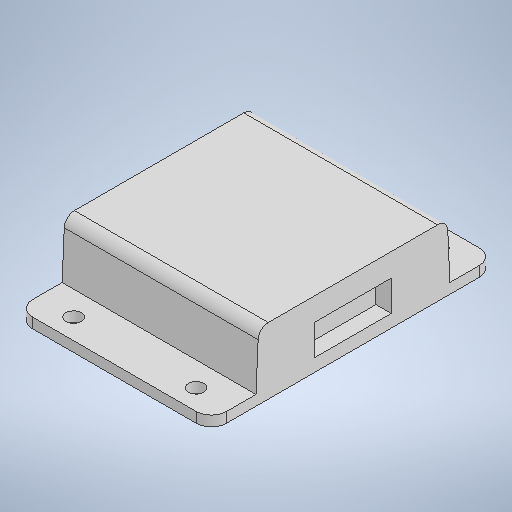
# Autodesk Inventor part: LiDAR_slave
Saved by Autodesk Inventor 2025.1 (Build 291241020, 241B)
## iProperties
Created: 2024-09-23
Part Number: LiDAR_slave
Material: 一般
Document SubType Name: Modeling
Designer: 8326d
Density: 1 g/cm^3
Appearance: 既定
Author: 8326d
Autodesk Inventor part; units mm, degrees
ref_plane "YZ Plane" through (0, 0, 0) normal (1, 0, 0) x (0, 1, 0)
ref_plane "XZ Plane" through (0, 0, 0) normal (0, 1, 0) x (-1, 0, 0)
ref_plane "XY Plane" through (0, 0, 0) normal (0, 0, 1) x (1, 0, 0)
sketch "スケッチ1" plane through (0, 0, 0) normal (1, 0, 0) x (0, 1, 0)
  line L0 (-6.5, 27.75) -> (6.5, 27.75)
  line L1 (6.5, 27.75) -> (6.5, -27.75)
  line L2 (6.5, -27.75) -> (-6.5, -27.75)
  line L3 (-6.5, -27.75) -> (-6.5, 27.75)
  line L4 (-6.5, 27.75) -> (6.5, -27.75) construction
  line L5 (6.5, 27.75) -> (-6.5, -27.75) construction
  line L6 (6.5, 19) -> (-4.5, 19)
  line L7 (-4.5, 19) -> (-4.5, -19)
  line L8 (-4.5, -19) -> (6.5, -19)
  line L9 (6.5, -19) -> (6.5, 19)
  line L10 (-4.5, 27.75) -> (-4.5, 19)
  line L11 (-4.5, 19) -> (6.5, 18.5)
  line L12 (6.5, -18.5) -> (-4.5, -19)
  line L13 (-4.5, -19) -> (-4.5, -27.75)
  point P0 (0, 0)
  point P1 (6.5, 0)
  point P2 (6.5, 18.5)
  dimension "d0" = 13
  dimension "d1" = 55.5
  dimension "d2" = 11
  dimension "d3" = 38
  dimension "d4" = 0.5
  dimension "d5" = 0.5
  constraints: 28 end point, 6 point on line, 4 midpoint, 4 parallel, 2 horizontal, 2 perpendicular, 1 collinear
  measures "d0" distance of L1.end L2.end
  measures "d1" distance of L0.end L1.end
  measures "d2" distance of L8.end L7.end
  measures "d3" distance of L7.end L6.end
  measures "d4" distance from line of L6 L11.end
  measures "d5" distance from line of L8 L12.start
extrude "押し出し1" add sketch "スケッチ1" along normal mid plane 38 contours L0 L10 L7 L13 L2 L3 | L11 L1 L12 L7
fillet "フィレット1" radius 2 2 edges at (0, 6.5, 18.5) (0, 6.5, -18.5)
sketch "スケッチ2" plane through (-19, -4.5, 27.75) normal (0, 1, 0) x (1, 0, 0)
  line L0 (7, 4) -> (31, 4) construction
  line L1 (7, 4) -> (31, 4) construction
  line L2 (0, 0) -> (38, 0) construction
  point P0 (19, 27.75)
  point P1 (19, 4)
  dimension "d9" = 24
  dimension "d10" = 0
  dimension "d11" = 4
  constraints: 4 end point, 2 coincident, 2 horizontal, 1 collinear, 1 midpoint, 1 vertical alignment
  measures "d9" distance of L0.start L0.end
  measures "d10" distance between parallel lines of L0 L1
  measures "d11" distance between parallel lines of L2 L0
hole "穴1" at (-12, -4.5, 23.75) at (12, -4.5, 23.75) direction (0, -1, 0) diameter 3 end through all
fillet "フィレット2" radius 3 2 edges at (19, -5.5, 27.75) (-19, -5.5, 27.75)
mirror "ミラー1" about plane through (0, 0, 0) normal (0, 0, 1) of "穴1", "フィレット2"
sketch "スケッチ3" plane through (19, 0, 0) normal (1, 0, 0) x (0, 0, -1)
  line L0 (-7.5, -4) -> (7.5, -4)
  line L1 (7.5, -4) -> (7.5, 2)
  line L2 (7.5, 2) -> (-7.5, 2)
  line L3 (-7.5, 2) -> (-7.5, -4)
  line L4 (-7.5, -4) -> (7.5, 2) construction
  line L5 (7.5, -4) -> (-7.5, 2) construction
  line L6 (-24.75, -6.5) -> (24.75, -6.5) projected
  point P0 (0, 0)
  point P1 (0, -1)
  dimension "d20" = 15
  dimension "d21" = 6
  dimension "d22" = 2.5
  constraints: 12 end point, 2 midpoint, 2 parallel, 1 horizontal, 1 perpendicular, 1 vertical alignment
  measures "d20" distance of L2.end L1.end
  measures "d21" distance of L1.end L0.end
  measures "d22" distance between parallel lines of L6 L0
extrude "押し出し2" cut sketch "スケッチ3" against normal blind 3
sketch "スケッチ4" plane through (-19, 0, 0) normal (-1, 0, 0) x (0, 0, 1)
  line L0 (5.5, -1.5) -> (11.5, -1.5) construction
  line L1 (5.5, -3) -> (11.5, -3)
  line L2 (11.5, 0) -> (5.5, 0)
  arc A0 (5.5, 0) -> (5.5, -3) centre (5.5, -1.5) ccw
  arc A1 (11.5, -3) -> (11.5, 0) centre (11.5, -1.5) ccw
  line L3 (8.5, -1.5) -> (14.5, -1.5) construction
  line L4 (-12, -2.5) -> (-5, -2.5)
  line L5 (-5, -2.5) -> (-5, 0)
  line L6 (-5, 0) -> (-12, 0)
  line L7 (-12, 0) -> (-12, -2.5)
  line L8 (-12, -2.5) -> (-5, 0) construction
  line L9 (-5, -2.5) -> (-12, 0) construction
  point P0 (0, 0)
  point P1 (-8.5, -1.25)
  point P2 (-8.5, 0)
  point P3 (8.5, 0)
  dimension "d25" = 3
  dimension "d26" = 0
  dimension "d27" = 3
  dimension "d28" = 7
  dimension "d29" = 2.5
  dimension "d30" = 8.5
  dimension "d31" = 8.5
  constraints: 22 end point, 5 midpoint, 4 point on circle, 4 tangent, 3 horizontal, 3 parallel, 2 centre point, 2 horizontal alignment, 1 collinear, 1 perpendicular
  measures "d25" distance of L3.start L0.end
  measures "d26" distance between parallel lines of L0 L3
  measures "d27" diameter of A1
  measures "d28" distance of L6.end L5.end
  measures "d29" distance of L5.end L4.end
  measures "d30" horizontal distance of point (0, 0) point (-8.5, -1.25)
  measures "d31" horizontal distance of point (0, 0) L3.start
extrude "押し出し3" cut sketch "スケッチ4" against normal blind 5
fillet "フィレット3" radius 0.3 2 edges at (-16.5, -2.5, -12) (-16.5, -2.5, -5)
fillet "フィレット4" radius 2 2 edges at (-16.5, 0, -12) (-16.5, 0, -5)
equation "\"d5\" = d4"
equation "\"d30\" = d31"
